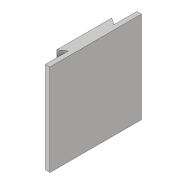
# Autodesk Inventor part: Sliding lock male test
Saved by Autodesk Inventor 2019 (Build 230136000, 136)
## iProperties
Created: 2019-10-09
Part Number: Sliding lock male test
Material: Generic
Document SubType Name: Modeling
Designer: ball
Density: 1 g/cm^3
Appearance: Default
Author: ball
Autodesk Inventor part; units mm, degrees
ref_plane "YZ Plane" through (0, 0, 0) normal (1, 0, 0) x (0, 1, 0)
ref_plane "XZ Plane" through (0, 0, 0) normal (0, 1, 0) x (-1, 0, 0)
ref_plane "XY Plane" through (0, 0, 0) normal (0, 0, 1) x (1, 0, 0)
sketch "Sketch1" plane through (0, 0, 0) normal (0, 1, 0) x (-1, 0, 0)
  line L0 (0, 0) -> (1.27, 0)
  line L1 (1.27, -25.4) -> (0, -25.4)
  line L2 (0, -25.4) -> (0, 0)
  line L3 (1.27, -6.35) -> (3.175, -6.35) construction
  line L4 (3.175, -6.35) -> (3.175, -19.05)
  line L5 (3.175, -19.05) -> (1.27, -19.05) construction
  line L6 (3.175, -19.05) -> (3.175, -20.32)
  line L7 (3.175, -20.32) -> (1.27, -19.05)
  line L8 (3.175, -6.35) -> (3.175, -5.08)
  line L9 (3.175, -5.08) -> (1.27, -6.35)
  line L10 (1.27, 0) -> (1.27, -6.35)
  line L11 (1.27, -19.05) -> (1.27, -25.4)
  dimension "d0" = 1.27
  dimension "d1" = 25.4
  dimension "d3" = 12.7
  dimension "d4" = 6.35
  dimension "d7" = 1.27
  dimension "d8" = 1.27
  constraints: 24 end point, 4 parallel, 3 perpendicular, 2 horizontal, 2 vertical
  measures "d0" distance of L1.start L1.end
  measures "d1" distance of L0.end L1.start
  measures "d3" distance of L3.end L4.end
  measures "d4" distance between parallel lines of L3 L0
  measures "d7" distance of L4.end L6.end
  measures "d8" distance of L3.end L8.end
extrude "Extrusion1" add sketch "Sketch1" along normal blind 25.4
body "Solid1"
